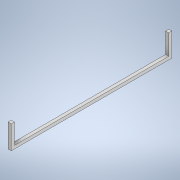
# Autodesk Inventor part: brace
Saved by Autodesk Inventor 2020.2 (Build 242310000, 310)
## iProperties
Created: 2020-02-12
Part Number: brace
Material: Generic
Document SubType Name: Modeling
Designer: ColinP
Density: 1 g/cm^3
Appearance: Default
Author: ColinP
Autodesk Inventor part; units mm, degrees
ref_plane "YZ Plane" through (0, 0, 0) normal (1, 0, 0) x (0, 1, 0)
ref_plane "XZ Plane" through (0, 0, 0) normal (0, 1, 0) x (-1, 0, 0)
ref_plane "XY Plane" through (0, 0, 0) normal (0, 0, 1) x (1, 0, 0)
sketch "Sketch1" plane through (0, 0, 0) normal (0, 1, 0) x (-1, 0, 0)
  line L0 (0, 0) -> (4, 0)
  line L1 (4, 0) -> (4, 197.612)
  line L2 (4, 197.612) -> (0, 197.612)
  line L3 (0, 197.612) -> (0, 0)
  line L4 (4, 197.612) -> (0, 197.612)
  line L5 (0, 197.612) -> (0, 201.612)
  line L6 (0, 201.612) -> (4, 201.612)
  line L7 (4, 201.612) -> (4, 197.612)
  line L8 (0, 0) -> (4, 0)
  line L9 (4, 0) -> (4, -4)
  line L10 (4, -4) -> (0, -4)
  line L11 (0, -4) -> (0, 0)
  dimension "d0" = 4
  dimension "d1" = 197.612
  dimension "d2" = 4
  dimension "d3" = 4
  dimension "d4" = 4
  dimension "d5" = 4
  constraints: 24 end point, 6 parallel, 3 horizontal, 3 perpendicular
  measures "d0" distance of L2.end L1.end
  measures "d1" distance of L1.end L0.end
  measures "d2" distance of L5.end L6.end
  measures "d3" distance of L4.end L5.end
  measures "d4" distance of L9.end L10.end
  measures "d5" distance of L8.end L9.end
extrude "Extrusion1" add sketch "Sketch1" along normal blind 30 contours L0 L9 L10 L11 | L5 L6 L7 L2
extrude "Extrusion2" add sketch "Sketch1" along normal blind 4 contours L3 L2 L1 L0
body "Solid1"
